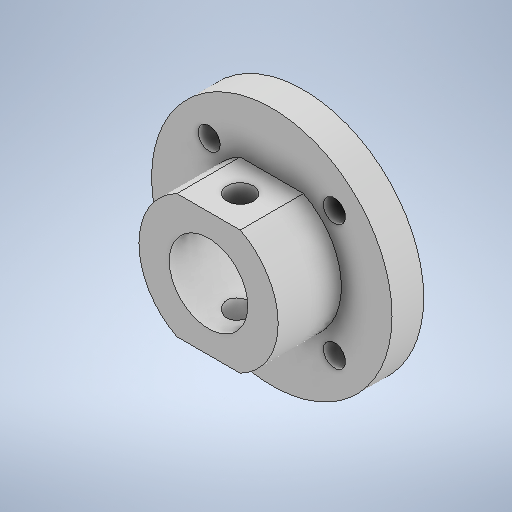
# Autodesk Inventor part: light_tire_fixer_10
Saved by Autodesk Inventor 2025.1 (Build 291241000, 241)
## iProperties
Created: 2024-12-20
Part Number: light_tire_fixer_10
Material: 一般
Document SubType Name: Modeling
Designer: yuki0520
Density: 1 g/cm^3
Appearance: 既定
Author: yuki0520
Autodesk Inventor part; units mm, degrees
ref_plane "YZ Plane" through (0, 0, 0) normal (1, 0, 0) x (0, 1, 0)
ref_plane "XZ Plane" through (0, 0, 0) normal (0, 1, 0) x (-1, 0, 0)
ref_plane "XY Plane" through (0, 0, 0) normal (0, 0, 1) x (1, 0, 0)
sketch "スケッチ1" plane through (0, 0, 0) normal (0, 0, 1) x (1, 0, 0)
  circle A0 centre (0, 0) radius 19
  circle A1 centre (0, 0) radius 14
  circle A2 centre (-14, 0) radius 1.75
  circle A3 centre (0, -14) radius 1.75
  circle A4 centre (14, 0) radius 1.75
  circle A5 centre (0, 14) radius 1.75
  line L0 (-19, 0) -> (19, 0)
  dimension "d10" = 28
  dimension "d0" = 38
  dimension "d11" = 3.5
  dimension "d14" = 360
  constraints: 5 centre point, 2 coincident, 2 end point, 2 point on circle, 1 horizontal, 1 horizontal alignment, 1 point on line, 11 other
  measures "d0" diameter of A0
  measures "d11" diameter of A2
extrude "押し出し1" add sketch "スケッチ1" along normal blind 5
sketch "スケッチ2" plane through (0, 0, 5) normal (0, 0, 1) x (1, 0, 0)
  circle A0 centre (0, 0) radius 11
  line L0 (5, -9.798) -> (-5, -9.798)
  line L1 (-5, -9.798) -> (-5, 9.798)
  line L2 (-5, 9.798) -> (5, 9.798)
  line L3 (5, 9.798) -> (5, -9.798)
  line L4 (5, -9.798) -> (-5, 9.798) construction
  line L5 (-5, -9.798) -> (5, 9.798) construction
  dimension "d3" = 22
  dimension "d6" = 10
  constraints: 12 end point, 2 midpoint, 2 parallel, 1 coincident, 1 horizontal, 1 perpendicular, 3 other
  measures "d6" distance of L1.end L2.end
extrude "押し出し2" add sketch "スケッチ2" along normal blind 10 contours A0 L3 | L3 L0 L1 L2 | L1 A0
sketch "スケッチ3" plane through (0, 0, 0) normal (0, 0, -1) x (-1, 0, 0)
  circle A0 centre (0, 0) radius 6.2
  dimension "d7" = 12.4
  constraints: 1 centre point, 1 coincident
  measures "d7" diameter of A0
extrude "押し出し3" cut sketch "スケッチ3" against normal blind 30
sketch "スケッチ4" plane through (0, 0, 0) normal (0, 0, -1) x (-1, 0, 0)
  circle A0 centre (0, 0) radius 14
  point P0 (-14, 0)
  point P1 (-9.8995, -9.8995)
  point P2 (0, -14)
  point P3 (9.8995, -9.8995)
  point P4 (14, 0)
  point P5 (9.8995, 9.8995)
  point P6 (0, 14)
  point P7 (-9.8995, 9.8995)
  dimension "d16" = 28
  dimension "d33" = 360
  constraints: 1 coincident, 1 horizontal alignment, 11 other
hole "穴1" at (9.8995, -9.8995, 0) at (9.8995, 9.8995, 0) at (-9.8995, 9.8995, 0) at (-9.8995, -9.8995, 0) direction (0, 0, 1) diameter 3.5 end through all
sketch "スケッチ5" plane through (-5, 9.798, 5) normal (0, 1, 0) x (1, 0, 0)
  line L0 (10, -10) -> (0, -10) projected
  line L1 (5, -10) -> (5, 0)
  line L2 (0, 0) -> (10, 0) projected
  point P0 (5, 5)
  point P1 (5, -5)
  constraints: 3 midpoint, 2 end point
hole "穴2" at (0, 9.798, 10) direction (0, -1, 0) diameter 4.2 end through all
